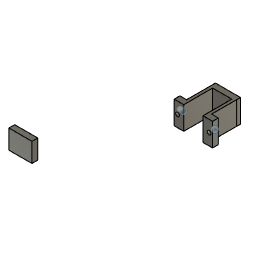
armMotorHolder (Autodesk Fusion 360 design; units mm, degrees)
Autodesk Fusion 360 part; units mm, degrees
sketch "Sketch1" plane through (0, 0, 0) normal (0, 0, 1) x (1, 0, 0)
  line L0 (15, 75) -> (25, 75)
  line L1 (25, 75) -> (25, 59)
  line L2 (25, 59) -> (15, 59)
  line L3 (15, 59) -> (15, 75)
  line L4 (15, 59) -> (11, 59)
  line L5 (11, 59) -> (11, 62)
  line L6 (11, 62) -> (15, 62)
  line L7 (15, 62) -> (15, 59)
  line L8 (25, 59) -> (29, 59)
  line L9 (29, 59) -> (29, 62)
  line L10 (29, 62) -> (25, 62)
  line L11 (25, 62) -> (25, 59)
  line L12 (15, 62) -> (13.5, 62)
  line L13 (13.5, 62) -> (13.5, 75)
  line L14 (13.5, 75) -> (15, 75)
  line L15 (15, 75) -> (15, 62)
  line L16 (25, 62) -> (26.5, 62)
  line L17 (26.5, 62) -> (26.5, 75)
  line L18 (26.5, 75) -> (25, 75)
  line L19 (25, 75) -> (25, 62)
  line L20 (13.5, 75) -> (26.543, 75)
  line L21 (26.543, 75) -> (26.543, 78)
  line L22 (26.543, 78) -> (13.5, 78)
  line L23 (13.5, 78) -> (13.5, 75)
  dimension "d2" = 10
  dimension "d3" = 16
  dimension "d4" = 4
  dimension "d5" = 3
  dimension "d6" = 4
  dimension "d7" = 3
  dimension "d8" = 1.5
  dimension "d9" = 1.5
  dimension "d10" = 3
  constraint horizontal L0
  constraint vertical L1
  constraint horizontal L2
  constraint vertical L3
  constraint horizontal L4
  constraint vertical L5
  constraint horizontal L6
  constraint vertical L7
  constraint horizontal L8
  constraint vertical L9
  constraint horizontal L10
  constraint vertical L11
  constraint horizontal L12
  constraint vertical L13
  constraint horizontal L14
  constraint vertical L15
  constraint horizontal L16
  constraint vertical L17
  constraint horizontal L18
  constraint vertical L19
  constraint horizontal L20
  constraint vertical L21
  constraint horizontal L22
  constraint vertical L23
  measures "d2" distance of L0.start L0.end
  measures "d3" distance of L0.start L2.end
  measures "d4" distance of L2.end L4.end
  measures "d5" distance of L2.end L6.end
  measures "d6" distance of L1.end L8.end
  measures "d7" distance of L1.end L10.end
  measures "d8" distance of L6.end L12.end
  measures "d9" distance of L10.end L16.end
  measures "d10" distance of L13.end L22.end
extrude "Extrude1" add sketch "Sketch1" along normal blind 12 contours L0 L14 L18 L20 L21 L22 L23 | L3 L6 L12 L13 L14 L15 L20 | L1 L10 L16 L17 L18 L19 L20 | L3 L4 L5 L6 L7 L12 | L1 L8 L9 L10 L11 L16 makes body 1
extrude "Extrude2" add 1 faces at (11, 60, 4) along direction (-1, 0, 0) blind 1 on bodies 1 bodies 1
extrude "Extrude3" add 1 faces at (29, 60, 4) along direction (1, 0, 0) blind 1 on bodies 1 bodies 1
sketch "Sketch2" plane through (0, 62, 0) normal (0, 1, 0) x (-1, 0, 0)
  line L0 (-30, 0) -> (-26.5, 0)
  line L1 (-26.5, 0) -> (-26.5, 12)
  line L2 (-26.5, 12) -> (-30, 12)
  line L3 (-30, 12) -> (-30, 0)
  circle A0 centre (-28.1976, 6) radius 1
  circle A1 centre (-28.1976, 6) radius 1
  line L4 (-28.1976, 6) -> (-30, 6)
  line L5 (-9.9996, 6) -> (-11.8016, 6)
  circle A2 centre (-11.8016, 6) radius 1
  dimension "d17" = 2
  dimension "d18" = 2
  dimension "d19" = 1.802
  dimension "d20" = 2
  constraint coincident A0.centre A1.centre
  constraint midpoint L3 L4.end
  constraint perpendicular L3 L4
  constraint perpendicular L3 L5
  constraint coincident L5.end A2.centre
  measures "d17" diameter of A0
  measures "d18" diameter of A1
  measures "d19" distance of L5.start L5.end
  measures "d20" diameter of A2
extrude "Extrude4" cut sketch "Sketch2" against normal blind 6 contours A2 bodies 1
extrude "Extrude5" cut sketch "Sketch2" against normal blind 5 contours A0 A1 bodies 1
box "BoxPrimitive1" add length 12 width 3 height 11 placed x (0, 0, -1) y (0, -1, 0) z (-1, 0, 0) at (25, 62, 12) bodies 1
extrude "Extrude6" add 1 faces at (18.3333, 75, 4) along direction (0, -1, 0) blind 1 on bodies 1 bodies 1
extrude "Extrude7" cut 1 faces at (22.1954, 78, 4) along direction (0, -1, 0) blind 1 on bodies 1 bodies 1
sketch "Sketch4" plane through (0, 0, 0) normal (0, 1, 0) x (1, 0, 0)
  line L0 (-5, -15) -> (-17, -15)
  line L1 (-17, -15) -> (-17, -5)
  line L2 (-17, -5) -> (-5, -5)
  line L3 (-5, -5) -> (-5, -15)
  dimension "d34" = 12
  dimension "d35" = 10
  constraint horizontal L0
  constraint vertical L1
  constraint horizontal L2
  constraint vertical L3
  measures "d34" distance of L0.start L0.end
  measures "d35" distance of L0.start L2.end
extrude "Extrude8" add sketch "Sketch4" along normal blind 3 separate body makes body 2
extrude "Extrude9" cut 1 faces at (21.6667, 62, 4) along direction (0, -1, 0) blind 3 on bodies 1 bodies 1
